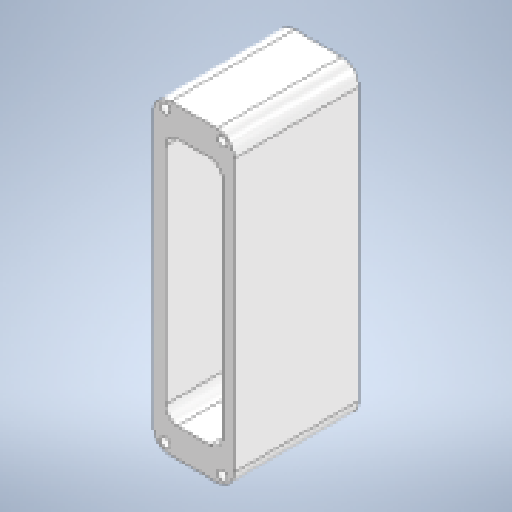
# Autodesk Inventor part: suzikai
Saved by Autodesk Inventor 2024 (Build 280153000, 153)
## iProperties
Created: 2023-12-16
Part Number: suzikai
Material: ABS プラスチック
Document SubType Name: Modeling
Designer: right
Mass: 13.6761 g
Surface Area: 75.438 cm^2
Volume: 12.902 cm^3
Density: 1.06 g/cm^3
Appearance: 滑らか - 白
Author: right
Autodesk Inventor part; units mm, degrees
ref_plane "YZ Plane" through (0, 0, 0) normal (1, 0, 0) x (0, 1, 0)
ref_plane "XZ Plane" through (0, 0, 0) normal (0, 1, 0) x (-1, 0, 0)
sketch "スケッチ1" plane through (0, 0, 0) normal (0, 0, 1) x (1, 0, 0)
  circle A0 centre (7, -1.5) radius 1.1 projected
  circle A1 centre (-7, -1.5) radius 1.1 projected
  arc A2 (-7, 6.5) -> (-4, 3.5) centre (-4, 6.5) ccw projected
  line L0 (4, 3.5) -> (-4, 3.5) projected
  arc A3 (4, 3.5) -> (7, 6.5) centre (4, 6.5) ccw projected
  line L1 (7, 27.5) -> (7, 6.5) projected
  line L2 (-7, 6.5) -> (-7, 27.5) projected
  arc A4 (-4, 30.5) -> (-7, 27.5) centre (-4, 27.5) ccw projected
  line L3 (-4, 30.5) -> (4, 30.5) projected
  circle A5 centre (-7, 35.5) radius 1.1 projected
  circle A6 centre (7, 35.5) radius 1.1 projected
  circle A7 centre (-7, -1.5) radius 1.1 projected
  line L4 (7, 27.5) -> (7, 6.5) projected
  arc A8 (4, 3.5) -> (7, 6.5) centre (4, 6.5) ccw projected
  line L5 (4, 3.5) -> (-4, 3.5) projected
  arc A9 (-7, 6.5) -> (-4, 3.5) centre (-4, 6.5) ccw projected
  line L6 (-7, 6.5) -> (-7, 27.5) projected
  arc A10 (-4, 30.5) -> (-7, 27.5) centre (-4, 27.5) ccw projected
  line L7 (-4, 30.5) -> (4, 30.5) projected
  arc A11 (7, 27.5) -> (4, 30.5) centre (4, 27.5) ccw projected
  circle A12 centre (7, -1.5) radius 1.1 projected
  arc A13 (6, -30) -> (6.4, -31.2) centre (8, -30) ccw projected
  arc A14 (6.4, -40.8) -> (6.4, -31.2) centre (0, -36) ccw projected
  arc A15 (6.4, -40.8) -> (6, -42) centre (8, -42) ccw projected
  line L8 (6, -42) -> (6, -42.5) projected
  arc A16 (6, -42.5) -> (10, -42.5) centre (8, -42.5) ccw projected
  line L9 (10, -42.5) -> (10, 76.5) projected
  arc A17 (10, 76.5) -> (6, 76.5) centre (8, 76.5) ccw projected
  line L10 (6, 76.5) -> (6, 76) projected
  arc A18 (6, 76) -> (6.4, 74.8) centre (8, 76) ccw projected
  arc A19 (6.4, 65.2) -> (6.4, 74.8) centre (0, 70) ccw projected
  arc A20 (6.4, 65.2) -> (6, 64) centre (8, 64) ccw projected
  line L11 (6, 64) -> (6, 60.696) projected
  arc A21 (6, 60.696) -> (6.9906, 58.9694) centre (8, 60.696) ccw projected
  line L12 (6.9906, 58.9694) -> (6.9906, 52.6121) projected
  arc A22 (6.9906, 52.6121) -> (6, 50.8855) centre (8, 50.8855) ccw projected
  line L13 (6, 50.8855) -> (6, 45.5) projected
  arc A23 (3, 42.5) -> (6, 45.5) centre (3, 45.5) ccw projected
  line L14 (3, 42.5) -> (-8, 42.5) projected
  arc A24 (-8, 42.5) -> (-10, 40.5) centre (-8, 40.5) ccw projected
  line L15 (-10, 40.5) -> (-10, -6.5) projected
  arc A25 (-10, -6.5) -> (-8, -8.5) centre (-8, -6.5) ccw projected
  line L16 (-8, -8.5) -> (3, -8.5) projected
  arc A26 (6, -11.5) -> (3, -8.5) centre (3, -11.5) ccw projected
  line L17 (6, -11.5) -> (6, -16.8855) projected
  arc A27 (6, -16.8855) -> (6.9906, -18.6121) centre (8, -16.8855) ccw projected
  line L18 (6.9906, -18.6121) -> (6.9906, -24.9694) projected
  arc A28 (6.9906, -24.9694) -> (6, -26.696) centre (8, -26.696) ccw projected
  line L19 (6, -26.696) -> (6, -30) projected
  circle A29 centre (8, 76.5) radius 1.1 projected
  circle A30 centre (-8, 40.5) radius 1.1 projected
  circle A31 centre (-8, -6.5) radius 1.1 projected
  circle A32 centre (8, -42.5) radius 1.1 projected
  circle A33 centre (8, -6.5) radius 1.1 projected
  circle A34 centre (8, 40.5) radius 1.1 projected
  line L20 (10, 37.6) -> (-10, 37.6)
  line L21 (10, 17) -> (-10, 17) construction
  line L22 (10, -3.6) -> (-10, -3.6)
  point P0 (0, 0)
  point P1 (-10, -3.6)
  point P2 (10, -3.6)
  dimension "d0" = 1
  constraints: 6 end point, 2 midpoint, 2 point on line, 2 symmetric about line, 1 horizontal
  measures "d0" distance edge to line of A6 L20
ref_plane "作業平面1" through (-10, -78.5, 30.5) normal (0, 0, -1) x (0, 1, 0)
extrude "押し出し1" add sketch "スケッチ1" along normal up to surface (30.5 mm away) contours L22 L15 L20 L9
fillet "フィレット1" radius 4.25 4 edges at (10, 37.6, 15.25) (-10, 37.6, 15.25) (10, -3.6, 15.25) (-10, -3.6, 15.25)
